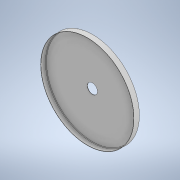
# Autodesk Inventor part: tapa_tambor
Saved by Autodesk Inventor 2021 (Build 250183000, 183)
## iProperties
Created: 2021-11-08
Part Number: tapa_tambor
Material: Genérico
Document SubType Name: Modeling
Designer: arthu
Density: 1 g/cm^3
Appearance: Valor por defecto
Author: arthu
Autodesk Inventor part; units mm, degrees
ref_plane "YZ Plane" through (0, 0, 0) normal (1, 0, 0) x (0, 1, 0)
ref_plane "XZ Plane" through (0, 0, 0) normal (0, 1, 0) x (-1, 0, 0)
ref_plane "XY Plane" through (0, 0, 0) normal (0, 0, 1) x (1, 0, 0)
sketch "Boceto1" plane through (0, 0, 0) normal (0, 0, 1) x (1, 0, 0)
  circle A0 centre (0, 0) radius 185
  circle A1 centre (0, 0) radius 183.8
  dimension "d0" = 370
  dimension "d1" = 367.6
  constraints: 2 centre point, 2 coincident
  measures "d0" diameter of A0
  measures "d1" diameter of A1
extrude "Extrusión1" add sketch "Boceto1" along normal blind 1.2 contours A1
extrude "Extrusión2" add sketch "Boceto1" along normal blind 21.2
fillet "Empalme1" radius 2 1 edges at (-183.8, 0, 1.2)
sketch "Boceto2" plane through (0, 0, 1.2) normal (0, 0, 1) x (1, 0, 0)
  circle A0 centre (0, 0) radius 20
  dimension "d7" = 40
  constraints: 1 centre point, 1 coincident
  measures "d7" diameter of A0
extrude "Extrusión3" cut sketch "Boceto2" against normal blind 10
